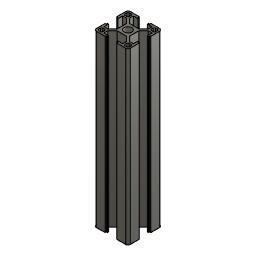
design2ver4 v30 (1) (Autodesk Fusion 360 archive; units mm, degrees)
design "Al profile 15 cm"
Autodesk Fusion 360 part; units mm, degrees
sketch "Sketch1" plane through (0, 0, 0) normal (0, 1, 0) x (1, 0, 0)
  line L0 (-13, 4.1) -> (-14, 4.1)
  line L1 (-12.5, 9.75) -> (-10.75, 9.75)
  line L2 (-13, 15) -> (-5.1, 15)
  line L3 (-10.75, 9.75) -> (-12.5, 9.75)
  line L4 (-8.25, 13) -> (-8.25, 9.6642)
  line L5 (-5.1, 15) -> (-13, 15)
  line L6 (-4.1, 13) -> (-8.25, 13)
  line L7 (-8.25, 9.6642) -> (-4.1, 5.5142)
  line L8 (-5.1, 14) -> (-4.1, 14)
  line L9 (-13, 8.25) -> (-9.6642, 8.25)
  line L10 (-8.25, 10.6606) -> (-8.25, 13)
  arc A0 (-13, 15) -> (-15, 13) centre (-13, 13) ccw
  line L11 (-9.75, 12.5) -> (-9.75, 10.75)
  arc A1 (-13.5, 10.75) -> (-12.5, 9.75) centre (-12.5, 10.75) ccw
  line L12 (-10.75, 13.5) -> (-12.5, 13.5)
  line L13 (-15, 13) -> (-15, 5.1)
  line L14 (-12.5, 13.5) -> (-10.75, 13.5)
  line L15 (-9.6642, 8.25) -> (-5.5142, 4.1)
  line L16 (-13, 8.25) -> (-13, 4.1)
  line L17 (-5.1, 14) -> (-5.1, 15)
  line L18 (13, -4.1) -> (14, -4.1)
  arc A2 (13.5, -10.75) -> (12.5, -9.75) centre (12.5, -10.75) ccw
  line L19 (8.25, -10.6606) -> (8.25, -13)
  line L20 (12.5, -9.75) -> (10.75, -9.75)
  arc A3 (13, -15) -> (15, -13) centre (13, -13) ccw
  circle A4 centre (0, 0) radius 3.4
  line L21 (14, -4.1) -> (14, -5.1)
  line L22 (12.5, -12.5) -> (-13, 13)
  line L23 (4.1, -13) -> (8.25, -13)
  line L24 (13, -4.1) -> (14, -4.1)
  line L25 (9.5009, 9.5009) -> (1.6153, 1.6153) construction
  line L26 (5.1, -14) -> (5.1, -15)
  line L27 (12.5, -13.5) -> (10.75, -13.5)
  line L28 (14, -5.1) -> (15, -5.1)
  arc A5 (9.75, -12.5) -> (10.75, -13.5) centre (10.75, -12.5) ccw
  line L29 (10.75, -9.75) -> (12.5, -9.75)
  line L30 (4.1, 5.5142) -> (-4.1, 5.5142)
  line L31 (13, -15) -> (5.1, -15)
  line L32 (15, -13) -> (15, -5.1)
  line L33 (8.25, -13) -> (8.25, -9.6642)
  line L34 (4.1, -5.5142) -> (-4.1, -5.5142)
  line L35 (13.5, -10.75) -> (13.5, -12.5)
  line L36 (4.1, -14) -> (4.1, -13)
  line L37 (5.1, -14) -> (4.1, -14)
  line L38 (5.1, -15) -> (13, -15)
  line L39 (5.5142, 4.1) -> (5.5142, -4.1)
  line L40 (9.6642, -8.25) -> (5.5142, -4.1)
  line L41 (15, -5.1) -> (15, -13)
  line L42 (9.75, -12.5) -> (9.75, -10.75)
  arc A6 (12.5, -13.5) -> (13.5, -12.5) centre (12.5, -12.5) ccw
  arc A7 (12.5, -13.5) -> (13.5, -12.5) centre (12.5, -12.5) ccw
  line L43 (13, -8.25) -> (13, -4.1)
  line L44 (8.25, 10.6606) -> (8.25, 13)
  line L45 (8.25, 13) -> (8.25, 9.6642)
  line L46 (-5.5142, 4.1) -> (-5.5142, -4.1)
  line L47 (-9.5009, -9.5009) -> (-1.6152, -1.6153) construction
  line L48 (5.1, 15) -> (13, 15)
  line L49 (13, 15) -> (5.1, 15)
  arc A8 (13.5, 12.5) -> (12.5, 13.5) centre (12.5, 12.5) ccw
  line L50 (-15, -5.1) -> (-15, -13)
  line L51 (5.1, 14) -> (4.1, 14)
  arc A9 (-10.75, 9.75) -> (-9.75, 10.75) centre (-10.75, 10.75) ccw
  line L52 (-13, 4.1) -> (-14, 4.1)
  line L53 (-9.5009, 9.5009) -> (-1.6152, 1.6153) construction
  line L54 (-14, 4.1) -> (-14, 5.1)
  line L55 (-4.1, 14) -> (-4.1, 13)
  arc A10 (-12.5, 13.5) -> (-13.5, 12.5) centre (-12.5, 12.5) ccw
  line L56 (-15, 5.1) -> (-15, 13)
  arc A11 (-9.75, 12.5) -> (-10.75, 13.5) centre (-10.75, 12.5) ccw
  line L57 (-14, 5.1) -> (-15, 5.1)
  arc A12 (-12.5, 13.5) -> (-13.5, 12.5) centre (-12.5, 12.5) ccw
  line L58 (-13.5, 10.75) -> (-13.5, 12.5)
  line L59 (-8.25, -13) -> (-8.25, -9.6642)
  line L60 (-9.6642, -8.25) -> (-5.5142, -4.1)
  line L61 (-4.1, -13) -> (-8.25, -13)
  arc A13 (-13.5, -12.5) -> (-12.5, -13.5) centre (-12.5, -12.5) ccw
  line L62 (-15, -13) -> (-15, -5.1)
  line L63 (-14, -4.1) -> (-14, -5.1)
  line L64 (-13, -8.25) -> (-9.6642, -8.25)
  line L65 (-13, -8.25) -> (-13, -4.1)
  line L66 (-5.1, -14) -> (-4.1, -14)
  line L67 (-12.5, -9.75) -> (-10.75, -9.75)
  line L68 (-8.25, -10.6606) -> (-8.25, -13)
  arc A14 (-9.75, -10.75) -> (-10.75, -9.75) centre (-10.75, -10.75) ccw
  arc A15 (-13.5, -12.5) -> (-12.5, -13.5) centre (-12.5, -12.5) ccw
  arc A16 (-15, -13) -> (-13, -15) centre (-13, -13) ccw
  line L69 (-5.1, -15) -> (-13, -15)
  line L70 (9.6642, 8.25) -> (5.5142, 4.1)
  line L71 (13.5, 10.75) -> (13.5, 12.5)
  line L72 (14, 5.1) -> (15, 5.1)
  arc A17 (13.5, 12.5) -> (12.5, 13.5) centre (12.5, 12.5) ccw
  line L73 (13, 4.1) -> (14, 4.1)
  line L74 (4.1, 14) -> (4.1, 13)
  line L75 (12.5, 9.75) -> (10.75, 9.75)
  line L76 (10.75, 13.5) -> (12.5, 13.5)
  line L77 (13, 4.1) -> (14, 4.1)
  arc A18 (9.75, 10.75) -> (10.75, 9.75) centre (10.75, 10.75) ccw
  line L78 (5.1, 14) -> (5.1, 15)
  line L79 (15, 13) -> (15, 5.1)
  arc A19 (15, 13) -> (13, 15) centre (13, 13) ccw
  arc A20 (10.75, -9.75) -> (9.75, -10.75) centre (10.75, -10.75) ccw
  line L80 (8.25, -9.6642) -> (4.1, -5.5142)
  line L81 (14, 4.1) -> (14, 5.1)
  line L82 (13, 8.25) -> (9.6642, 8.25)
  line L83 (13, -8.25) -> (9.6642, -8.25)
  line L84 (9.5009, -9.5009) -> (1.6153, -1.6153) construction
  line L85 (10.75, 9.75) -> (12.5, 9.75)
  line L86 (8.25, 9.6642) -> (4.1, 5.5142)
  line L87 (15, 5.1) -> (15, 13)
  line L88 (13, 8.25) -> (13, 4.1)
  line L89 (12.5, 13.5) -> (10.75, 13.5)
  arc A21 (10.75, 13.5) -> (9.75, 12.5) centre (10.75, 12.5) ccw
  line L90 (10.75, -13.5) -> (12.5, -13.5)
  line L91 (4.1, 13) -> (8.25, 13)
  line L92 (9.75, 12.5) -> (9.75, 10.75)
  arc A22 (12.5, 9.75) -> (13.5, 10.75) centre (12.5, 10.75) ccw
  line L93 (-14, -5.1) -> (-15, -5.1)
  line L94 (-13, -15) -> (-5.1, -15)
  line L95 (-4.1, -14) -> (-4.1, -13)
  arc A23 (-12.5, -9.75) -> (-13.5, -10.75) centre (-12.5, -10.75) ccw
  line L96 (-10.75, -9.75) -> (-12.5, -9.75)
  line L97 (-12.5, -13.5) -> (-10.75, -13.5)
  line L98 (-8.25, -9.6642) -> (-4.1, -5.5142)
  line L99 (-13.5, -10.75) -> (-13.5, -12.5)
  arc A24 (-10.75, -13.5) -> (-9.75, -12.5) centre (-10.75, -12.5) ccw
  line L100 (-5.1, -14) -> (-5.1, -15)
  line L101 (-13, -4.1) -> (-14, -4.1)
  line L102 (-10.75, -13.5) -> (-12.5, -13.5)
  line L103 (-13, -4.1) -> (-14, -4.1)
  line L104 (-9.75, -12.5) -> (-9.75, -10.75)
  point P0 (-15, -15)
  point P1 (-14, -4.1)
  point P2 (-15, 0)
  point P3 (-5.1, -14)
  point P4 (-5.1, 14)
  point P5 (-12.5, -12.5)
  point P6 (-14, -5.1)
  point P7 (0, 0)
  point P8 (-15, -5.1)
  point P9 (-13, -8.25)
  point P10 (0, 0)
  point P11 (0, 15)
  point P12 (15, 15)
  point P13 (12.5, 12.5)
  point P14 (5.1, 15)
  point P15 (15, 0)
  point P16 (0, 0)
  point P17 (5.1, 14)
  point P18 (14, 4.1)
  point P19 (13, 8.25)
  point P20 (-12.5, 12.5)
  point P21 (8.25, 13)
  point P22 (-8.25, 13)
  point P23 (14, 5.1)
  point P24 (4.1, 14)
  point P25 (15, 5.1)
  point P26 (-15, 0)
  point P27 (-4.1, 13)
  point P28 (-5.1, 15)
  point P29 (4.1, 13)
  point P30 (-5.1, -15)
  point P31 (0, -15)
  point P32 (0, 0)
  point P33 (0, 15)
  point P34 (-4.1, 14)
  point P35 (-13, 8.25)
  point P36 (0, 0)
  point P37 (-4.1, -14)
  point P38 (0, 15)
  point P39 (-4.1, -13)
  point P40 (-14, 4.1)
  point P41 (-15, 5.1)
  point P42 (-14, 5.1)
  point P43 (0, 0)
  point P44 (-8.25, -13)
  point P45 (-15, 15)
  point P46 (5.1, -15)
  point P47 (15, -15)
  point P48 (4.1, -14)
  point P49 (15, -5.1)
  point P50 (13, -8.25)
  point P51 (4.1, -13)
  point P52 (14, -4.1)
  point P53 (5.1, -14)
  point P54 (8.25, -13)
  point P55 (14, -5.1)
  dimension "d1" = 2
  dimension "d2" = 1
  dimension "d3" = 1.5
  dimension "d4" = 1
  dimension "d5" = 1
  dimension "d6" = 1.5
  dimension "d7" = 1.5
  dimension "d8" = 1.5
  dimension "d9" = 8.2
  dimension "d10" = 8.2
  dimension "d11" = 6.8
  constraint coincident L18.start L24.start
  constraint coincident P52 L18.end
  constraint coincident P55 L21.end
  constraint coincident P49 L28.end
  constraint coincident P46 L26.end
  constraint coincident P53 L26.start
  constraint coincident P48 L36.start
  constraint coincident P51 L23.start
  constraint coincident P54 L19.end
  constraint tangent A3 L41
  constraint tangent A3 L31
  constraint horizontal L27
  constraint vertical L42
  constraint horizontal L29
  constraint vertical L35
  constraint tangent L35 A6
  constraint tangent L27 A6
  constraint tangent L27 A5
  constraint tangent A5 L42
  constraint equal A5 A6
  constraint tangent L42 A20
  constraint tangent L29 A20
  constraint equal A6 A20
  constraint tangent A2 L29
  constraint tangent A2 L35
  constraint equal A2 A6
  constraint coincident L84.start L22
  constraint coincident L84.end L22
  constraint parallel L22 L84
  constraint perpendicular L23 L33
  constraint coincident P50 L43.start
  constraint perpendicular L43 L83
  constraint parallel L40 L84
  constraint parallel L80 L84
  constraint perpendicular L26 L31
  constraint coincident P43 P36
  measures "d1" radius of A3
  measures "d2" radius of A6
  measures "d3" distance of L32 L35
  measures "d4" distance of L40 L84
  measures "d5" distance of L22 L80
  measures "d6" distance of L33 L42
  measures "d7" distance of L29 L83
  measures "d8" distance of L27 L31
  measures "d9" distance of L34.end L34.start
  measures "d10" distance of L39.end L39.start
  measures "d11" diameter of A4
extrude "Extrude1" add sketch "Sketch1" along normal blind 150

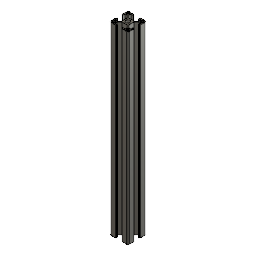
design "Al profile 30 cm"
Autodesk Fusion 360 part; units mm, degrees
sketch "Sketch1" plane through (0, 0, 0) normal (0, 1, 0) x (1, 0, 0)
  line L0 (-13, 4.1) -> (-14, 4.1)
  line L1 (-12.5, 9.75) -> (-10.75, 9.75)
  line L2 (-13, 15) -> (-5.1, 15)
  line L3 (-10.75, 9.75) -> (-12.5, 9.75)
  line L4 (-8.25, 13) -> (-8.25, 9.6642)
  line L5 (-5.1, 15) -> (-13, 15)
  line L6 (-4.1, 13) -> (-8.25, 13)
  line L7 (-8.25, 9.6642) -> (-4.1, 5.5142)
  line L8 (-5.1, 14) -> (-4.1, 14)
  line L9 (-13, 8.25) -> (-9.6642, 8.25)
  line L10 (-8.25, 10.6606) -> (-8.25, 13)
  arc A0 (-13, 15) -> (-15, 13) centre (-13, 13) ccw
  line L11 (-9.75, 12.5) -> (-9.75, 10.75)
  arc A1 (-13.5, 10.75) -> (-12.5, 9.75) centre (-12.5, 10.75) ccw
  line L12 (-10.75, 13.5) -> (-12.5, 13.5)
  line L13 (-15, 13) -> (-15, 5.1)
  line L14 (-12.5, 13.5) -> (-10.75, 13.5)
  line L15 (-9.6642, 8.25) -> (-5.5142, 4.1)
  line L16 (-13, 8.25) -> (-13, 4.1)
  line L17 (-5.1, 14) -> (-5.1, 15)
  line L18 (13, -4.1) -> (14, -4.1)
  arc A2 (13.5, -10.75) -> (12.5, -9.75) centre (12.5, -10.75) ccw
  line L19 (8.25, -10.6606) -> (8.25, -13)
  line L20 (12.5, -9.75) -> (10.75, -9.75)
  arc A3 (13, -15) -> (15, -13) centre (13, -13) ccw
  circle A4 centre (0, 0) radius 3.4
  line L21 (14, -4.1) -> (14, -5.1)
  line L22 (12.5, -12.5) -> (-13, 13)
  line L23 (4.1, -13) -> (8.25, -13)
  line L24 (13, -4.1) -> (14, -4.1)
  line L25 (9.5009, 9.5009) -> (1.6153, 1.6153) construction
  line L26 (5.1, -14) -> (5.1, -15)
  line L27 (12.5, -13.5) -> (10.75, -13.5)
  line L28 (14, -5.1) -> (15, -5.1)
  arc A5 (9.75, -12.5) -> (10.75, -13.5) centre (10.75, -12.5) ccw
  line L29 (10.75, -9.75) -> (12.5, -9.75)
  line L30 (4.1, 5.5142) -> (-4.1, 5.5142)
  line L31 (13, -15) -> (5.1, -15)
  line L32 (15, -13) -> (15, -5.1)
  line L33 (8.25, -13) -> (8.25, -9.6642)
  line L34 (4.1, -5.5142) -> (-4.1, -5.5142)
  line L35 (13.5, -10.75) -> (13.5, -12.5)
  line L36 (4.1, -14) -> (4.1, -13)
  line L37 (5.1, -14) -> (4.1, -14)
  line L38 (5.1, -15) -> (13, -15)
  line L39 (5.5142, 4.1) -> (5.5142, -4.1)
  line L40 (9.6642, -8.25) -> (5.5142, -4.1)
  line L41 (15, -5.1) -> (15, -13)
  line L42 (9.75, -12.5) -> (9.75, -10.75)
  arc A6 (12.5, -13.5) -> (13.5, -12.5) centre (12.5, -12.5) ccw
  arc A7 (12.5, -13.5) -> (13.5, -12.5) centre (12.5, -12.5) ccw
  line L43 (13, -8.25) -> (13, -4.1)
  line L44 (8.25, 10.6606) -> (8.25, 13)
  line L45 (8.25, 13) -> (8.25, 9.6642)
  line L46 (-5.5142, 4.1) -> (-5.5142, -4.1)
  line L47 (-9.5009, -9.5009) -> (-1.6152, -1.6153) construction
  line L48 (5.1, 15) -> (13, 15)
  line L49 (13, 15) -> (5.1, 15)
  arc A8 (13.5, 12.5) -> (12.5, 13.5) centre (12.5, 12.5) ccw
  line L50 (-15, -5.1) -> (-15, -13)
  line L51 (5.1, 14) -> (4.1, 14)
  arc A9 (-10.75, 9.75) -> (-9.75, 10.75) centre (-10.75, 10.75) ccw
  line L52 (-13, 4.1) -> (-14, 4.1)
  line L53 (-9.5009, 9.5009) -> (-1.6152, 1.6153) construction
  line L54 (-14, 4.1) -> (-14, 5.1)
  line L55 (-4.1, 14) -> (-4.1, 13)
  arc A10 (-12.5, 13.5) -> (-13.5, 12.5) centre (-12.5, 12.5) ccw
  line L56 (-15, 5.1) -> (-15, 13)
  arc A11 (-9.75, 12.5) -> (-10.75, 13.5) centre (-10.75, 12.5) ccw
  line L57 (-14, 5.1) -> (-15, 5.1)
  arc A12 (-12.5, 13.5) -> (-13.5, 12.5) centre (-12.5, 12.5) ccw
  line L58 (-13.5, 10.75) -> (-13.5, 12.5)
  line L59 (-8.25, -13) -> (-8.25, -9.6642)
  line L60 (-9.6642, -8.25) -> (-5.5142, -4.1)
  line L61 (-4.1, -13) -> (-8.25, -13)
  arc A13 (-13.5, -12.5) -> (-12.5, -13.5) centre (-12.5, -12.5) ccw
  line L62 (-15, -13) -> (-15, -5.1)
  line L63 (-14, -4.1) -> (-14, -5.1)
  line L64 (-13, -8.25) -> (-9.6642, -8.25)
  line L65 (-13, -8.25) -> (-13, -4.1)
  line L66 (-5.1, -14) -> (-4.1, -14)
  line L67 (-12.5, -9.75) -> (-10.75, -9.75)
  line L68 (-8.25, -10.6606) -> (-8.25, -13)
  arc A14 (-9.75, -10.75) -> (-10.75, -9.75) centre (-10.75, -10.75) ccw
  arc A15 (-13.5, -12.5) -> (-12.5, -13.5) centre (-12.5, -12.5) ccw
  arc A16 (-15, -13) -> (-13, -15) centre (-13, -13) ccw
  line L69 (-5.1, -15) -> (-13, -15)
  line L70 (9.6642, 8.25) -> (5.5142, 4.1)
  line L71 (13.5, 10.75) -> (13.5, 12.5)
  line L72 (14, 5.1) -> (15, 5.1)
  arc A17 (13.5, 12.5) -> (12.5, 13.5) centre (12.5, 12.5) ccw
  line L73 (13, 4.1) -> (14, 4.1)
  line L74 (4.1, 14) -> (4.1, 13)
  line L75 (12.5, 9.75) -> (10.75, 9.75)
  line L76 (10.75, 13.5) -> (12.5, 13.5)
  line L77 (13, 4.1) -> (14, 4.1)
  arc A18 (9.75, 10.75) -> (10.75, 9.75) centre (10.75, 10.75) ccw
  line L78 (5.1, 14) -> (5.1, 15)
  line L79 (15, 13) -> (15, 5.1)
  arc A19 (15, 13) -> (13, 15) centre (13, 13) ccw
  arc A20 (10.75, -9.75) -> (9.75, -10.75) centre (10.75, -10.75) ccw
  line L80 (8.25, -9.6642) -> (4.1, -5.5142)
  line L81 (14, 4.1) -> (14, 5.1)
  line L82 (13, 8.25) -> (9.6642, 8.25)
  line L83 (13, -8.25) -> (9.6642, -8.25)
  line L84 (9.5009, -9.5009) -> (1.6153, -1.6153) construction
  line L85 (10.75, 9.75) -> (12.5, 9.75)
  line L86 (8.25, 9.6642) -> (4.1, 5.5142)
  line L87 (15, 5.1) -> (15, 13)
  line L88 (13, 8.25) -> (13, 4.1)
  line L89 (12.5, 13.5) -> (10.75, 13.5)
  arc A21 (10.75, 13.5) -> (9.75, 12.5) centre (10.75, 12.5) ccw
  line L90 (10.75, -13.5) -> (12.5, -13.5)
  line L91 (4.1, 13) -> (8.25, 13)
  line L92 (9.75, 12.5) -> (9.75, 10.75)
  arc A22 (12.5, 9.75) -> (13.5, 10.75) centre (12.5, 10.75) ccw
  line L93 (-14, -5.1) -> (-15, -5.1)
  line L94 (-13, -15) -> (-5.1, -15)
  line L95 (-4.1, -14) -> (-4.1, -13)
  arc A23 (-12.5, -9.75) -> (-13.5, -10.75) centre (-12.5, -10.75) ccw
  line L96 (-10.75, -9.75) -> (-12.5, -9.75)
  line L97 (-12.5, -13.5) -> (-10.75, -13.5)
  line L98 (-8.25, -9.6642) -> (-4.1, -5.5142)
  line L99 (-13.5, -10.75) -> (-13.5, -12.5)
  arc A24 (-10.75, -13.5) -> (-9.75, -12.5) centre (-10.75, -12.5) ccw
  line L100 (-5.1, -14) -> (-5.1, -15)
  line L101 (-13, -4.1) -> (-14, -4.1)
  line L102 (-10.75, -13.5) -> (-12.5, -13.5)
  line L103 (-13, -4.1) -> (-14, -4.1)
  line L104 (-9.75, -12.5) -> (-9.75, -10.75)
  point P0 (-15, -15)
  point P1 (-14, -4.1)
  point P2 (-15, 0)
  point P3 (-5.1, -14)
  point P4 (-5.1, 14)
  point P5 (-12.5, -12.5)
  point P6 (-14, -5.1)
  point P7 (0, 0)
  point P8 (-15, -5.1)
  point P9 (-13, -8.25)
  point P10 (0, 0)
  point P11 (0, 15)
  point P12 (15, 15)
  point P13 (12.5, 12.5)
  point P14 (5.1, 15)
  point P15 (15, 0)
  point P16 (0, 0)
  point P17 (5.1, 14)
  point P18 (14, 4.1)
  point P19 (13, 8.25)
  point P20 (-12.5, 12.5)
  point P21 (8.25, 13)
  point P22 (-8.25, 13)
  point P23 (14, 5.1)
  point P24 (4.1, 14)
  point P25 (15, 5.1)
  point P26 (-15, 0)
  point P27 (-4.1, 13)
  point P28 (-5.1, 15)
  point P29 (4.1, 13)
  point P30 (-5.1, -15)
  point P31 (0, -15)
  point P32 (0, 0)
  point P33 (0, 15)
  point P34 (-4.1, 14)
  point P35 (-13, 8.25)
  point P36 (0, 0)
  point P37 (-4.1, -14)
  point P38 (0, 15)
  point P39 (-4.1, -13)
  point P40 (-14, 4.1)
  point P41 (-15, 5.1)
  point P42 (-14, 5.1)
  point P43 (0, 0)
  point P44 (-8.25, -13)
  point P45 (-15, 15)
  point P46 (5.1, -15)
  point P47 (15, -15)
  point P48 (4.1, -14)
  point P49 (15, -5.1)
  point P50 (13, -8.25)
  point P51 (4.1, -13)
  point P52 (14, -4.1)
  point P53 (5.1, -14)
  point P54 (8.25, -13)
  point P55 (14, -5.1)
  dimension "d1" = 2
  dimension "d2" = 1
  dimension "d3" = 1.5
  dimension "d4" = 1
  dimension "d5" = 1
  dimension "d6" = 1.5
  dimension "d7" = 1.5
  dimension "d8" = 1.5
  dimension "d9" = 8.2
  dimension "d10" = 8.2
  dimension "d11" = 6.8
  constraint coincident L18.start L24.start
  constraint coincident P52 L18.end
  constraint coincident P55 L21.end
  constraint coincident P49 L28.end
  constraint coincident P46 L26.end
  constraint coincident P53 L26.start
  constraint coincident P48 L36.start
  constraint coincident P51 L23.start
  constraint coincident P54 L19.end
  constraint tangent A3 L41
  constraint tangent A3 L31
  constraint horizontal L27
  constraint vertical L42
  constraint horizontal L29
  constraint vertical L35
  constraint tangent L35 A6
  constraint tangent L27 A6
  constraint tangent L27 A5
  constraint tangent A5 L42
  constraint equal A5 A6
  constraint tangent L42 A20
  constraint tangent L29 A20
  constraint equal A6 A20
  constraint tangent A2 L29
  constraint tangent A2 L35
  constraint equal A2 A6
  constraint coincident L84.start L22
  constraint coincident L84.end L22
  constraint parallel L22 L84
  constraint perpendicular L23 L33
  constraint coincident P50 L43.start
  constraint perpendicular L43 L83
  constraint parallel L40 L84
  constraint parallel L80 L84
  constraint perpendicular L26 L31
  constraint coincident P43 P36
  measures "d1" radius of A3
  measures "d2" radius of A6
  measures "d3" distance of L32 L35
  measures "d4" distance of L40 L84
  measures "d5" distance of L22 L80
  measures "d6" distance of L33 L42
  measures "d7" distance of L29 L83
  measures "d8" distance of L27 L31
  measures "d9" distance of L34.end L34.start
  measures "d10" distance of L39.end L39.start
  measures "d11" diameter of A4
extrude "Extrude1" add sketch "Sketch1" along normal blind 300

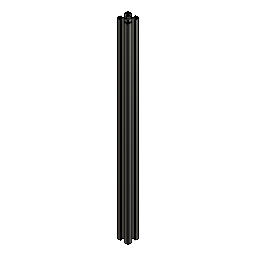
design "Al profile 50 cm"
Autodesk Fusion 360 part; units mm, degrees
sketch "Sketch1" plane through (0, 0, 0) normal (0, 1, 0) x (1, 0, 0)
  line L0 (-13, 4.1) -> (-14, 4.1)
  line L1 (-12.5, 9.75) -> (-10.75, 9.75)
  line L2 (-13, 15) -> (-5.1, 15)
  line L3 (-10.75, 9.75) -> (-12.5, 9.75)
  line L4 (-8.25, 13) -> (-8.25, 9.6642)
  line L5 (-5.1, 15) -> (-13, 15)
  line L6 (-4.1, 13) -> (-8.25, 13)
  line L7 (-8.25, 9.6642) -> (-4.1, 5.5142)
  line L8 (-5.1, 14) -> (-4.1, 14)
  line L9 (-13, 8.25) -> (-9.6642, 8.25)
  line L10 (-8.25, 10.6606) -> (-8.25, 13)
  arc A0 (-13, 15) -> (-15, 13) centre (-13, 13) ccw
  line L11 (-9.75, 12.5) -> (-9.75, 10.75)
  arc A1 (-13.5, 10.75) -> (-12.5, 9.75) centre (-12.5, 10.75) ccw
  line L12 (-10.75, 13.5) -> (-12.5, 13.5)
  line L13 (-15, 13) -> (-15, 5.1)
  line L14 (-12.5, 13.5) -> (-10.75, 13.5)
  line L15 (-9.6642, 8.25) -> (-5.5142, 4.1)
  line L16 (-13, 8.25) -> (-13, 4.1)
  line L17 (-5.1, 14) -> (-5.1, 15)
  line L18 (13, -4.1) -> (14, -4.1)
  arc A2 (13.5, -10.75) -> (12.5, -9.75) centre (12.5, -10.75) ccw
  line L19 (8.25, -10.6606) -> (8.25, -13)
  line L20 (12.5, -9.75) -> (10.75, -9.75)
  arc A3 (13, -15) -> (15, -13) centre (13, -13) ccw
  circle A4 centre (0, 0) radius 3.4
  line L21 (14, -4.1) -> (14, -5.1)
  line L22 (12.5, -12.5) -> (-13, 13)
  line L23 (4.1, -13) -> (8.25, -13)
  line L24 (13, -4.1) -> (14, -4.1)
  line L25 (9.5009, 9.5009) -> (1.6153, 1.6153) construction
  line L26 (5.1, -14) -> (5.1, -15)
  line L27 (12.5, -13.5) -> (10.75, -13.5)
  line L28 (14, -5.1) -> (15, -5.1)
  arc A5 (9.75, -12.5) -> (10.75, -13.5) centre (10.75, -12.5) ccw
  line L29 (10.75, -9.75) -> (12.5, -9.75)
  line L30 (4.1, 5.5142) -> (-4.1, 5.5142)
  line L31 (13, -15) -> (5.1, -15)
  line L32 (15, -13) -> (15, -5.1)
  line L33 (8.25, -13) -> (8.25, -9.6642)
  line L34 (4.1, -5.5142) -> (-4.1, -5.5142)
  line L35 (13.5, -10.75) -> (13.5, -12.5)
  line L36 (4.1, -14) -> (4.1, -13)
  line L37 (5.1, -14) -> (4.1, -14)
  line L38 (5.1, -15) -> (13, -15)
  line L39 (5.5142, 4.1) -> (5.5142, -4.1)
  line L40 (9.6642, -8.25) -> (5.5142, -4.1)
  line L41 (15, -5.1) -> (15, -13)
  line L42 (9.75, -12.5) -> (9.75, -10.75)
  arc A6 (12.5, -13.5) -> (13.5, -12.5) centre (12.5, -12.5) ccw
  arc A7 (12.5, -13.5) -> (13.5, -12.5) centre (12.5, -12.5) ccw
  line L43 (13, -8.25) -> (13, -4.1)
  line L44 (8.25, 10.6606) -> (8.25, 13)
  line L45 (8.25, 13) -> (8.25, 9.6642)
  line L46 (-5.5142, 4.1) -> (-5.5142, -4.1)
  line L47 (-9.5009, -9.5009) -> (-1.6152, -1.6153) construction
  line L48 (5.1, 15) -> (13, 15)
  line L49 (13, 15) -> (5.1, 15)
  arc A8 (13.5, 12.5) -> (12.5, 13.5) centre (12.5, 12.5) ccw
  line L50 (-15, -5.1) -> (-15, -13)
  line L51 (5.1, 14) -> (4.1, 14)
  arc A9 (-10.75, 9.75) -> (-9.75, 10.75) centre (-10.75, 10.75) ccw
  line L52 (-13, 4.1) -> (-14, 4.1)
  line L53 (-9.5009, 9.5009) -> (-1.6152, 1.6153) construction
  line L54 (-14, 4.1) -> (-14, 5.1)
  line L55 (-4.1, 14) -> (-4.1, 13)
  arc A10 (-12.5, 13.5) -> (-13.5, 12.5) centre (-12.5, 12.5) ccw
  line L56 (-15, 5.1) -> (-15, 13)
  arc A11 (-9.75, 12.5) -> (-10.75, 13.5) centre (-10.75, 12.5) ccw
  line L57 (-14, 5.1) -> (-15, 5.1)
  arc A12 (-12.5, 13.5) -> (-13.5, 12.5) centre (-12.5, 12.5) ccw
  line L58 (-13.5, 10.75) -> (-13.5, 12.5)
  line L59 (-8.25, -13) -> (-8.25, -9.6642)
  line L60 (-9.6642, -8.25) -> (-5.5142, -4.1)
  line L61 (-4.1, -13) -> (-8.25, -13)
  arc A13 (-13.5, -12.5) -> (-12.5, -13.5) centre (-12.5, -12.5) ccw
  line L62 (-15, -13) -> (-15, -5.1)
  line L63 (-14, -4.1) -> (-14, -5.1)
  line L64 (-13, -8.25) -> (-9.6642, -8.25)
  line L65 (-13, -8.25) -> (-13, -4.1)
  line L66 (-5.1, -14) -> (-4.1, -14)
  line L67 (-12.5, -9.75) -> (-10.75, -9.75)
  line L68 (-8.25, -10.6606) -> (-8.25, -13)
  arc A14 (-9.75, -10.75) -> (-10.75, -9.75) centre (-10.75, -10.75) ccw
  arc A15 (-13.5, -12.5) -> (-12.5, -13.5) centre (-12.5, -12.5) ccw
  arc A16 (-15, -13) -> (-13, -15) centre (-13, -13) ccw
  line L69 (-5.1, -15) -> (-13, -15)
  line L70 (9.6642, 8.25) -> (5.5142, 4.1)
  line L71 (13.5, 10.75) -> (13.5, 12.5)
  line L72 (14, 5.1) -> (15, 5.1)
  arc A17 (13.5, 12.5) -> (12.5, 13.5) centre (12.5, 12.5) ccw
  line L73 (13, 4.1) -> (14, 4.1)
  line L74 (4.1, 14) -> (4.1, 13)
  line L75 (12.5, 9.75) -> (10.75, 9.75)
  line L76 (10.75, 13.5) -> (12.5, 13.5)
  line L77 (13, 4.1) -> (14, 4.1)
  arc A18 (9.75, 10.75) -> (10.75, 9.75) centre (10.75, 10.75) ccw
  line L78 (5.1, 14) -> (5.1, 15)
  line L79 (15, 13) -> (15, 5.1)
  arc A19 (15, 13) -> (13, 15) centre (13, 13) ccw
  arc A20 (10.75, -9.75) -> (9.75, -10.75) centre (10.75, -10.75) ccw
  line L80 (8.25, -9.6642) -> (4.1, -5.5142)
  line L81 (14, 4.1) -> (14, 5.1)
  line L82 (13, 8.25) -> (9.6642, 8.25)
  line L83 (13, -8.25) -> (9.6642, -8.25)
  line L84 (9.5009, -9.5009) -> (1.6153, -1.6153) construction
  line L85 (10.75, 9.75) -> (12.5, 9.75)
  line L86 (8.25, 9.6642) -> (4.1, 5.5142)
  line L87 (15, 5.1) -> (15, 13)
  line L88 (13, 8.25) -> (13, 4.1)
  line L89 (12.5, 13.5) -> (10.75, 13.5)
  arc A21 (10.75, 13.5) -> (9.75, 12.5) centre (10.75, 12.5) ccw
  line L90 (10.75, -13.5) -> (12.5, -13.5)
  line L91 (4.1, 13) -> (8.25, 13)
  line L92 (9.75, 12.5) -> (9.75, 10.75)
  arc A22 (12.5, 9.75) -> (13.5, 10.75) centre (12.5, 10.75) ccw
  line L93 (-14, -5.1) -> (-15, -5.1)
  line L94 (-13, -15) -> (-5.1, -15)
  line L95 (-4.1, -14) -> (-4.1, -13)
  arc A23 (-12.5, -9.75) -> (-13.5, -10.75) centre (-12.5, -10.75) ccw
  line L96 (-10.75, -9.75) -> (-12.5, -9.75)
  line L97 (-12.5, -13.5) -> (-10.75, -13.5)
  line L98 (-8.25, -9.6642) -> (-4.1, -5.5142)
  line L99 (-13.5, -10.75) -> (-13.5, -12.5)
  arc A24 (-10.75, -13.5) -> (-9.75, -12.5) centre (-10.75, -12.5) ccw
  line L100 (-5.1, -14) -> (-5.1, -15)
  line L101 (-13, -4.1) -> (-14, -4.1)
  line L102 (-10.75, -13.5) -> (-12.5, -13.5)
  line L103 (-13, -4.1) -> (-14, -4.1)
  line L104 (-9.75, -12.5) -> (-9.75, -10.75)
  point P0 (-15, -15)
  point P1 (-14, -4.1)
  point P2 (-15, 0)
  point P3 (-5.1, -14)
  point P4 (-5.1, 14)
  point P5 (-12.5, -12.5)
  point P6 (-14, -5.1)
  point P7 (0, 0)
  point P8 (-15, -5.1)
  point P9 (-13, -8.25)
  point P10 (0, 0)
  point P11 (0, 15)
  point P12 (15, 15)
  point P13 (12.5, 12.5)
  point P14 (5.1, 15)
  point P15 (15, 0)
  point P16 (0, 0)
  point P17 (5.1, 14)
  point P18 (14, 4.1)
  point P19 (13, 8.25)
  point P20 (-12.5, 12.5)
  point P21 (8.25, 13)
  point P22 (-8.25, 13)
  point P23 (14, 5.1)
  point P24 (4.1, 14)
  point P25 (15, 5.1)
  point P26 (-15, 0)
  point P27 (-4.1, 13)
  point P28 (-5.1, 15)
  point P29 (4.1, 13)
  point P30 (-5.1, -15)
  point P31 (0, -15)
  point P32 (0, 0)
  point P33 (0, 15)
  point P34 (-4.1, 14)
  point P35 (-13, 8.25)
  point P36 (0, 0)
  point P37 (-4.1, -14)
  point P38 (0, 15)
  point P39 (-4.1, -13)
  point P40 (-14, 4.1)
  point P41 (-15, 5.1)
  point P42 (-14, 5.1)
  point P43 (0, 0)
  point P44 (-8.25, -13)
  point P45 (-15, 15)
  point P46 (5.1, -15)
  point P47 (15, -15)
  point P48 (4.1, -14)
  point P49 (15, -5.1)
  point P50 (13, -8.25)
  point P51 (4.1, -13)
  point P52 (14, -4.1)
  point P53 (5.1, -14)
  point P54 (8.25, -13)
  point P55 (14, -5.1)
  dimension "d1" = 2
  dimension "d2" = 1
  dimension "d3" = 1.5
  dimension "d4" = 1
  dimension "d5" = 1
  dimension "d6" = 1.5
  dimension "d7" = 1.5
  dimension "d8" = 1.5
  dimension "d9" = 8.2
  dimension "d10" = 8.2
  dimension "d11" = 6.8
  constraint coincident L18.start L24.start
  constraint coincident P52 L18.end
  constraint coincident P55 L21.end
  constraint coincident P49 L28.end
  constraint coincident P46 L26.end
  constraint coincident P53 L26.start
  constraint coincident P48 L36.start
  constraint coincident P51 L23.start
  constraint coincident P54 L19.end
  constraint tangent A3 L41
  constraint tangent A3 L31
  constraint horizontal L27
  constraint vertical L42
  constraint horizontal L29
  constraint vertical L35
  constraint tangent L35 A6
  constraint tangent L27 A6
  constraint tangent L27 A5
  constraint tangent A5 L42
  constraint equal A5 A6
  constraint tangent L42 A20
  constraint tangent L29 A20
  constraint equal A6 A20
  constraint tangent A2 L29
  constraint tangent A2 L35
  constraint equal A2 A6
  constraint coincident L84.start L22
  constraint coincident L84.end L22
  constraint parallel L22 L84
  constraint perpendicular L23 L33
  constraint coincident P50 L43.start
  constraint perpendicular L43 L83
  constraint parallel L40 L84
  constraint parallel L80 L84
  constraint perpendicular L26 L31
  constraint coincident P43 P36
  measures "d1" radius of A3
  measures "d2" radius of A6
  measures "d3" distance of L32 L35
  measures "d4" distance of L40 L84
  measures "d5" distance of L22 L80
  measures "d6" distance of L33 L42
  measures "d7" distance of L29 L83
  measures "d8" distance of L27 L31
  measures "d9" distance of L34.end L34.start
  measures "d10" distance of L39.end L39.start
  measures "d11" diameter of A4
extrude "Extrude1" add sketch "Sketch1" along normal blind 500
